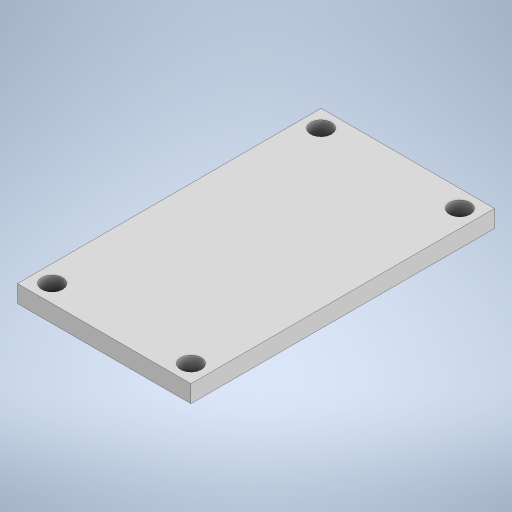
# Autodesk Inventor part: 0_mm_slant
Saved by Autodesk Inventor 2023.1 (Build 271208000, 208)
## iProperties
Created: 2023-05-29
Part Number: 0_mm_slant
Material: Generic
Document SubType Name: Modeling
Designer: Mansoor Lunawadi
Density: 1 g/cm^3
Appearance: Default
Author: Mansoor Lunawadi
Autodesk Inventor part; units mm, degrees
ref_plane "YZ Plane" through (0, 0, 0) normal (1, 0, 0) x (0, 1, 0)
ref_plane "XZ Plane" through (0, 0, 0) normal (0, 1, 0) x (-1, 0, 0)
ref_plane "XY Plane" through (0, 0, 0) normal (0, 0, 1) x (1, 0, 0)
sketch "Sketch1" plane through (0, 0, 0) normal (1, 0, 0) x (0, 1, 0)
  line L0 (0, 0) -> (2, 0)
  line L1 (0, 0) -> (0, -35)
  line L2 (2, 0) -> (2, -35)
  line L3 (2, -35) -> (0, -35)
  dimension "d0" = 2
  dimension "d1" = 35
  constraints: 8 end point, 1 horizontal, 1 parallel, 1 perpendicular, 1 vertical
  measures "d0" distance of L0.start L0.end
  measures "d1" distance of L0.start L1.end
extrude "Extrusion1" add sketch "Sketch1" along normal blind 20
sketch "Sketch2" plane through (0, 0, -35) normal (0, -1, 0) x (1, 0, 0)
  line L0 (0, 35) -> (20, 35) projected
  circle A0 centre (18, 33) radius 1.2
  line L1 (0, 35) -> (0, 0) projected
  circle A1 centre (2, 33) radius 1.2
  line L2 (20, 35) -> (20, 0) projected
  circle A2 centre (18, 2) radius 1.2
  circle A3 centre (2, 2) radius 1.2
  dimension "d6" = 2.4
  dimension "d8" = 2.4
  dimension "d12" = 2.4
  dimension "d13" = 2.4
  constraints: 4 centre point
  measures "d6" diameter of A0
  measures "d8" diameter of A1
  measures "d12" diameter of A2
  measures "d13" diameter of A3
extrude "Extrusion2" cut sketch "Sketch2" against normal through all
body "Solid1"
